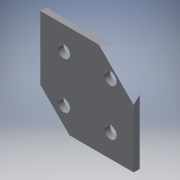
# Autodesk Inventor part: fly wheel gusset
Saved by Autodesk Inventor 2016 (Build 200138000, 138)
## iProperties
Created: 2016-02-03
Part Number: fly wheel gusset
Material: Aluminum 6061
Document SubType Name: Modeling
Designer: gus
Density: 2.7 g/cm^3
Appearance: Aluminum - Flat
Mass: 31.9579 g
Surface Area: 85.3155 cm^2
Volume: 11.8363 cm^3
Author: gus
Autodesk Inventor part; units mm, degrees
ref_plane "YZ Plane" through (0, 0, 0) normal (1, 0, 0) x (0, 1, 0)
ref_plane "XZ Plane" through (0, 0, 0) normal (0, 1, 0) x (-1, 0, 0)
ref_plane "XY Plane" through (0, 0, 0) normal (0, 0, 1) x (1, 0, 0)
sketch "Sketch1" plane through (0, 0, 0) normal (0, 0, 1) x (1, 0, 0)
  line L0 (0, 0) -> (-50.8, 0)
  line L1 (-50.8, 0) -> (-50.8, 25.4)
  line L2 (-50.8, 25.4) -> (-50.8, 76.2)
  line L3 (-50.8, 76.2) -> (0, 76.2)
  line L4 (0, 76.2) -> (0, 0)
  circle A0 centre (-38.1, 12.7) radius 3.3734
  circle A1 centre (-12.7, 38.1) radius 3.3734
  circle A2 centre (-12.7, 63.5) radius 3.3734
  circle A3 centre (-38.1, 63.5) radius 3.3734
  dimension "d0" = 50.8
  dimension "d1" = 25.4
  dimension "d2" = 76.2
  dimension "d3" = 50.8
  dimension "d4" = 6.7469
  dimension "d5" = 38.1
  dimension "d6" = 12.7
  dimension "d7" = 38.1
  dimension "d9" = 12.7
  dimension "d10" = 12.7
  dimension "d14" = 12.7
  dimension "d15" = 12.7
  dimension "d18" = 12.7
  constraints: 10 end point, 4 centre point, 3 equal radius, 2 horizontal, 2 vertical
  measures "d0" distance of L0.start L0.end
  measures "d1" distance of L0.end L1.end
  measures "d2" distance of L3.end L0.start
  measures "d3" distance of L2.end L3.end
  measures "d4" diameter of A0
  measures "d5" distance from line of L0 A1.centre
  measures "d6" distance from line of L1 A0.centre
  measures "d7" distance from line of L1 A1.centre
  measures "d9" distance from line of L3 A3.centre
  measures "d10" distance from line of L3 A2.centre
  measures "d14" distance from line of L2 A3.centre
  measures "d15" distance from line of L4 A2.centre
  measures "d18" distance from line of L0 A0.centre
extrude "Extrusion2" add sketch "Sketch1" along normal blind 3.175
body "Solid2"
